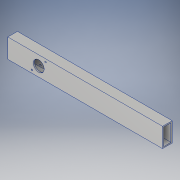
# Autodesk Inventor part: liftCimBar
Saved by Autodesk Inventor 2019 (Build 230136000, 136)
## iProperties
Created: 2019-01-15
Part Number: liftCimBar
Material: Aluminum 6061
Document SubType Name: Modeling
Designer: lebraddock
Density: 2.7 g/cm^3
Appearance: Aluminum - Flat
Mass: 464.203 g
Surface Area: 1105 cm^2
Volume: 171.927 cm^3
Author: lebraddock
Autodesk Inventor part; units mm, degrees
ref_plane "YZ Plane" through (0, 0, 0) normal (1, 0, 0) x (0, 1, 0)
ref_plane "XZ Plane" through (0, 0, 0) normal (0, 1, 0) x (-1, 0, 0)
ref_plane "XY Plane" through (0, 0, 0) normal (0, 0, 1) x (1, 0, 0)
sketch "Sketch1" plane through (0, 0, 0) normal (1, 0, 0) x (0, 1, 0)
  line L0 (0, 0) -> (50.8, 0)
  line L1 (50.8, 0) -> (50.8, -25.4)
  line L2 (50.8, -25.4) -> (0, -25.4)
  line L3 (0, -25.4) -> (0, 0)
  line L4 (47.625, -22.225) -> (47.625, -3.175)
  line L5 (47.625, -3.175) -> (3.175, -3.175)
  line L6 (3.175, -3.175) -> (3.175, -22.225)
  line L7 (3.175, -22.225) -> (47.625, -22.225)
  dimension "d0" = 50.8
  dimension "d1" = 25.4
  dimension "d2" = 3.175
  constraints: 16 end point, 4 parallel, 2 perpendicular, 1 horizontal, 3 other
  measures "d0" distance of L1.end L2.end
  measures "d1" distance of L0.end L1.end
  measures "d2" distance between parallel lines of L1 L4
extrude "Extrusion1" add sketch "Sketch1" along normal blind 177.8
sketch "Sketch2" plane through (0, 0, 0) normal (0, 0, 1) x (1, 0, 0)
  line L0 (0, 0) -> (0, 50.8) projected
  circle A0 centre (81.28, 25.4) radius 14.2875
  line L1 (151.13, 25.4) -> (175.8823, 25.4) construction
  line L2 (81.28, 25.4) -> (106.68, 25.4) construction
  circle A1 centre (99.2405, 43.3605) radius 2.0193
  circle A2 centre (63.3195, 7.4395) radius 2.0193
  circle A3 centre (63.3195, 7.4395) radius 2.0193
  circle A4 centre (99.2405, 43.3605) radius 2.0193
  dimension "d5" = 81.28
  dimension "d6" = 28.575
  dimension "d19" = 4.0386
  dimension "d20" = 4.0386
  constraints: 5 centre point, 4 end point, 3 coincident, 2 concentric, 2 horizontal
  measures "d5" distance from line of L0 A0.centre
  measures "d6" diameter of A0
  measures "d19" diameter of A1
  measures "d20" diameter of A2
extrude "Extrusion2" cut sketch "Sketch2" against normal blind 25.4 contours A0
sketch "Sketch3" plane through (177.8, 0, 0) normal (1, 0, 0) x (0, 0, -1)
  line L0 (0, 50.8) -> (0, 0) projected
  line L1 (25.4, 0) -> (25.4, 50.8) projected
  line L2 (0, 0) -> (25.4, 0)
  line L3 (25.4, 0) -> (25.4, 50.8)
  line L4 (25.4, 50.8) -> (0, 50.8)
  line L5 (0, 50.8) -> (0, 0)
  line L6 (3.175, 3.175) -> (3.175, 47.625) projected
  line L7 (3.175, 47.625) -> (22.225, 47.625) projected
  line L8 (3.175, 3.175) -> (22.225, 3.175)
  line L9 (22.225, 3.175) -> (22.225, 47.625)
  line L10 (22.225, 47.625) -> (3.175, 47.625)
  line L11 (3.175, 47.625) -> (3.175, 3.175)
  constraints: 16 end point, 4 parallel, 2 horizontal, 2 perpendicular
extrude "Extrusion3" add sketch "Sketch3" along normal blind 228.6
sketch "Sketch4" plane through (0, 0, 0) normal (0, 0, 1) x (1, 0, 0)
  circle A0 centre (81.28, 25.4) radius 14.2875 projected
  line L0 (0, 50.8) -> (406.4, 50.8) projected
  line L1 (81.28, 25.4) -> (106.68, 25.4) construction
  circle A1 centre (99.2405, 43.3605) radius 2.0193
  circle A2 centre (63.3195, 7.4395) radius 2.0193
  point P0 (0, 0)
  dimension "d22" = 4.0386
  dimension "d23" = 4.0386
  constraints: 2 centre point, 2 end point, 1 coincident, 1 horizontal
  measures "d22" diameter of A1
  measures "d23" diameter of A2
extrude "Extrusion4" cut sketch "Sketch4" against normal blind 228.6 contours A1 | A2
body "Solid1"
